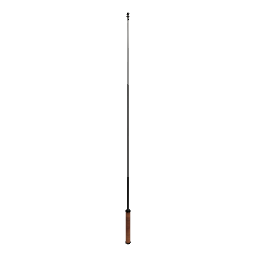
cat toy v3 (Autodesk Fusion 360 design; units mm, degrees)
Autodesk Fusion 360 part; units mm, degrees
note: some values were not read from the file. Chosen so that the rebuilt part matches the saved one: a setting.
sketch "base of handle" plane through (0, 0, 0) normal (0, 0, 1) x (1, 0, 0)
  circle A0 centre (0, 0) radius 7.25
  dimension "d1" = 14.5
  constraint coincident A0.centre origin
  measures "d1" diameter of A0
extrude "Extrude1" add sketch "base of handle" along normal blind 121 makes body 1
fillet "Fillet1" radius 0.5 1 edges at (-6.7594, -2.6217, 121) on bodies 1
fillet "Fillet2" radius 1 1 edges at (-6.7594, -2.6217, 0) on bodies 1
sketch "base of plastic part" plane through (0, 0, 121) normal (0, 0, 1) x (-1, 0, 0)
  circle A0 centre (0, 0) radius 6.75
  circle A1 centre (0, 0) radius 3
  dimension "d8" = 6
  constraint coincident A0.centre A1.centre
  measures "d8" diameter of A1
ref_plane "WorkPlane1" through (0, 0, 846) normal (0, 0, 1) x (-1, 0, 0)
sketch "top of plastic part" plane through (0, 0, 846) normal (0, 0, 1) x (1, 0, 0)
  circle A0 centre (0, 0) radius 1.4
  dimension "d10" = 2.8
  constraint coincident A0.centre origin
  measures "d10" diameter of A0
loft "Loft1" add profiles "base of plastic part", "top of plastic part" section 1 contours A1 section 2 bodies 1
sketch "centerpoint" plane through (0, 0, 0) normal (0, 1, 0) x (1, 0, 0)
  line L0 (0, -121) -> (0, -122.45) construction
  dimension "d11" = 1.45
  constraint vertical L0
  measures "d11" distance of L0.start L0.end
ref_plane "WorkPlane2" through (0, 0, 122.45) normal (0, 0, 1) x (1, 0, 0)
torus "TorusPrimitive2" add centre line diameter 9 section diameter 2.9 placed x (1, 0, 0) y (0, 1, 0) z (0, 0, 1) at (0, 0, 122.45) separate body makes body 2
sketch "Sketch7" plane through (0, 0, 0) normal (0, 1, 0) x (1, 0, 0)
  line L0 (-0.007, -848.5003) -> (2.243, -848.5003) construction
  line L1 (-0.007, -848.5003) -> (-0.007, -856.5003) construction
  line L2 (-0.007, -856.5003) -> (2.243, -856.5003) construction
  line L3 (-0.007, -856.5003) -> (-0.007, -858.5003) construction
  line L4 (-0.007, -858.5003) -> (2.993, -858.5003) construction
  line L5 (-0.007, -858.5003) -> (-0.007, -867.0003) construction
  line L6 (-0.007, -867.0003) -> (2.993, -867.0003) construction
  line L7 (1.693, -846.0003) -> (2.243, -848.5003)
  line L8 (2.243, -848.5003) -> (2.243, -856.5003)
  line L9 (2.243, -856.5003) -> (2.993, -858.5003)
  line L10 (2.993, -858.5003) -> (2.993, -867.0003)
  line L11 (1.493, -869.5003) -> (2.993, -867.0003)
  line L12 (0, -846) -> (1.693, -846.0003)
  line L13 (1.493, -869.5003) -> (0, -869.5003)
  line L14 (0, -869.5003) -> (0, -846)
  dimension "d26" = 2.25
  dimension "d27" = 8
  dimension "d28" = 2.25
  dimension "d29" = 2
  dimension "d30" = 3
  dimension "d31" = 8.5
  constraint perpendicular L0 L1
  constraint perpendicular L1 L2
  constraint perpendicular L2 L3
  constraint perpendicular L3 L4
  constraint perpendicular L4 L5
  constraint perpendicular L5 L6
  constraint equal L4 L6
  constraint horizontal L13
  constraint vertical L14
  measures "d26" distance of L0.start L0.end
  measures "d27" distance of L0.start L1.end
  measures "d28" distance of L1.end L2.end
  measures "d29" distance of L1.end L3.end
  measures "d30" distance of L3.end L4.end
  measures "d31" distance of L3.end L5.end
revolve "Revolve1" add sketch "Sketch7" angle 360 about axis through (0, 0, 1.75) along (0, 0, 1) separate body makes body 3
fillet "Fillet3" radius 0.05 1 edges at (-1.5784, -0.6122, 846.0003) on bodies 3
copy_body "CutPasteBodies1" bodies 1 removing the originals makes body 4 in component "fishing rod toy"
copy_body "CutPasteBodies2" bodies 2 removing the originals makes body 5 in component "fishing rod toy"
copy_body "CutPasteBodies3" bodies 3 removing the originals makes body 6 in component "fishing rod toy"
component "fishing rod toy" placed x (1, 0, 0) y (0, 1, 0) z (0, 0, 1) at (0, 0, 0)
equation "d11 = ( 2.9 / 2 ) * 1 mm"
equation "d14 = ( 2.9 / 2 ) * 1 mm"
equation "d_sec_2 = 4.5 mm"
equation "h_sec_1 = 2.5 mm"
equation "h_sec_2 = 8 mm"
equation "d_sec_4 = 6 mm"
equation "h_sec_3 = 2 mm"
equation "h_sec_4 = 8.5 mm"
equation "d_sec_5 = 3 mm"
equation "h_sec_5 = 2.5 mm"
equation "d26 = d_sec_2 / 2"
equation "d27 = h_sec_2"
equation "d28 = d_sec_2 / 2"
equation "d29 = h_sec_3"
equation "d30 = d_sec_4 / 2"
equation "d31 = h_sec_4"
